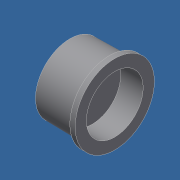
# Autodesk Inventor part: P1704_017_button_cap
Saved by Autodesk Inventor 2019 (Build 230136000, 136)
## iProperties
Created: 2019-05-23
Part Number: P1704_017_button_cap
Project: Nom Projet
Material: .
Description: Nom pièce
Document SubType Name: Modeling
Designer: Adel.KAHRIMANOVIC
Authority: brut Ø
Density: 0.001 g/cm^3
Appearance: Par défaut
Material number: ---
Author: Adel.KAHRIMANOVIC
Autodesk Inventor part; units mm, degrees
ref_plane "Plan YZ" through (0, 0, 0) normal (1, 0, 0) x (0, 1, 0)
ref_plane "Plan XZ" through (0, 0, 0) normal (0, 1, 0) x (-1, 0, 0)
ref_plane "Plan XY" through (0, 0, 0) normal (0, 0, 1) x (1, 0, 0)
sketch "Esquisse1" plane through (0, 0, 0) normal (0, 0, 1) x (1, 0, 0)
  line L0 (-11.0568, 0) -> (3.3738, 0)
  line L1 (-6.8, 5.2) -> (-0.8, 5.3)
  line L2 (-0.8, 5.3) -> (-0.8, 6)
  line L3 (-0.8, 6) -> (0, 6)
  line L4 (0, 6) -> (0, 0)
  line L5 (-7.5, 0) -> (0, 0)
  arc A0 (-6.8, 5.2) -> (-7.5, 0) centre (12.1643, 0) ccw
  line L6 (-15.701, 0) -> (16.8085, 0) construction
  line L7 (0, -1.2) -> (0, 7.2) construction
  point P0 (0, 0)
  dimension "d0" = 10.4
  dimension "d1" = 10.6
  dimension "d2" = 6
  dimension "d3" = 0.8
  dimension "d4" = 7.5
  dimension "d5" = 12
  constraints: 12 end point, 4 perpendicular, 3 point on circle, 2 collinear, 2 point on line, 1 centre point, 1 horizontal, 1 line through centre
  measures "d0" diameter of L1.start L0
  measures "d1" diameter of L1.end L0
  measures "d2" horizontal distance of L1.start L1.end
  measures "d3" distance of L2.end L3.end
  measures "d4" distance of L5.start L4.end
  measures "d5" diameter of L3 L0
revolve "Révolution1" add sketch "Esquisse1" angle 360 about axis through (-11.0568, 0, 0) along (1, 0, 0)
sketch "Esquisse6" plane through (0, 0, 0) normal (1, 0, 0) x (0, 0, -1)
  circle A0 centre (0, 0) radius 4.3
  dimension "d7" = 8.6
  constraints: 1 centre point, 1 coincident
  measures "d7" diameter of A0
extrude "Extrusion1" cut sketch "Esquisse6" against normal blind 3.4
